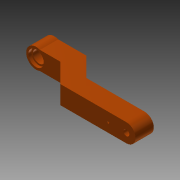
# Autodesk Inventor part: xy forearm
Saved by Autodesk Inventor 2013 (Build 170138000, 138)
## iProperties
Created: 2013-08-04
Part Number: xy forearm
Material: Generic
Document SubType Name: Modeling
Designer: employee
Density: 1 g/cm^3
Mass: 104.531 g
Surface Area: 212.692 cm^2
Volume: 104.531 cm^3
Author: employee
Autodesk Inventor part; units mm, degrees
ref_plane "YZ Plane" through (0, 0, 0) normal (1, 0, 0) x (0, 1, 0)
ref_plane "XZ Plane" through (0, 0, 0) normal (0, 1, 0) x (-1, 0, 0)
ref_plane "XY Plane" through (0, 0, 0) normal (0, 0, 1) x (1, 0, 0)
sketch "Sketch1" plane through (0, 0, 0) normal (0, 1, 0) x (-1, 0, 0)
  circle A0 centre (0, 0) radius 4.05
  line L0 (0, 12.5) -> (150, 12.5)
  arc A1 (150, -12.5) -> (150, 12.5) centre (150, 0) ccw
  line L1 (150, -12.5) -> (0, -12.5)
  arc A2 (0, 12.5) -> (0, -12.5) centre (0, 0) ccw
  dimension "d0" = 150
  dimension "d2" = 12.5
  dimension "d3" = 8.1
  constraints: 4 end point, 4 point on circle, 4 tangent, 3 centre point, 2 coincident, 1 horizontal, 1 parallel
  measures "d0" distance of A1.centre A2.centre
  measures "d2" radius of A2
  measures "d3" diameter of A0
extrude "Extrusion1" add sketch "Sketch1" along normal blind 25
sketch "Sketch2" plane through (0, 25, 0) normal (0, 1, 0) x (1, 0, 0)
  circle A0 centre (0, 0) radius 4.05 projected
  line L0 (-150, -12.5) -> (0, -12.5) projected
  line L1 (0, 12.5) -> (-150, 12.5) projected
  arc A1 (-150, 12.5) -> (-150, -12.5) centre (-150, 0) ccw projected
  line L2 (-80, 12.5) -> (-80, -12.5)
  dimension "d6" = 80
  constraints: 2 end point, 2 point on line, 1 perpendicular
  measures "d6" distance from line of A0.centre L2
extrude "Extrusion2" add sketch "Sketch2" along normal blind 26.5 contours A1 L1 L2 L0
sketch "Sketch3" plane through (-150, 0, 12.5) normal (0, 0, 1) x (1, 0, 0)
  line L0 (150, 0) -> (0, 0) projected
  line L1 (70, 25) -> (70, 51.5) projected
  line L2 (0, 51.5) -> (70, 51.5) projected
  line L3 (70, 25) -> (43.5, 51.5)
  line L4 (59.6447, 0) -> (33.1447, 26.5)
  line L5 (70, 51.5) -> (70, 25) projected
  line L6 (70, 25) -> (150, 25) projected
  line L7 (150, 0) -> (150, 25) projected
  line L8 (150, 0) -> (0, 0) projected
  line L9 (0, 0) -> (0, 51.5) projected
  line L10 (-12.5, 0) -> (-12.5, 51.5) projected
  line L11 (-12.5, 26.5) -> (33.1447, 26.5)
  line L12 (-12.5, 26.5) -> (-12.5, 0)
  line L13 (59.6447, 0) -> (-12.5, 0)
  line L14 (0, 51.5) -> (70, 51.5) projected
  dimension "d9" = 45
  dimension "d10" = 25
  dimension "d11" = 25
  constraints: 10 end point, 3 point on line, 2 collinear, 1 parallel, 1 perpendicular
  measures "d9" angle of L1 L3
  measures "d10" distance between parallel lines of L3 L4
  measures "d11" distance from line of L2.start L11
extrude "Extrusion3" cut sketch "Sketch3" against normal through all contours L0 L9 L11 L4 | L13 L10 L11 L9
sketch "Sketch4" plane through (0, 0, 12.5) normal (0, 0, 1) x (1, 0, 0)
  line L0 (-116.8553, 26.5) -> (-90.3553, 0) projected
  line L1 (-80, 25) -> (-80, 51.5) projected
  line L2 (-150, 51.5) -> (-80, 51.5) projected
  line L3 (-80, 25) -> (-106.5, 51.5)
  constraints: 2 end point, 1 parallel, 1 point on line
extrude "Extrusion4" cut sketch "Sketch4" against normal through all
sketch "Sketch5" plane through (0, 51.5, 0) normal (0, 1, 0) x (1, 0, 0)
  arc A0 (-150, 12.5) -> (-150, -12.5) centre (-150, 0) ccw projected
  circle A1 centre (-150, 0) radius 8.3
  point P0 (0, 0)
  dimension "d20" = 16.6
  constraints: 1 centre point, 1 coincident
  measures "d20" diameter of A1
extrude "Extrusion5" cut sketch "Sketch5" against normal through all
sketch "Sketch6" plane through (0, 51.5, 0) normal (0, 1, 0) x (1, 0, 0)
  circle A0 centre (-150, 0) radius 8.3 projected
  arc A1 (-150, 12.5) -> (-150, -12.5) centre (-150, 0) ccw projected
  circle A2 centre (-150, 0) radius 10.55
  point P0 (0, 0)
  dimension "d26" = 21.1
  constraints: 1 centre point, 1 coincident
  measures "d26" diameter of A2
extrude "Extrusion6" cut sketch "Sketch6" against normal blind 4
sketch "Sketch7" plane through (-150, 26.5, 12.5) normal (0, -1, 0) x (1, 0, 0)
  circle A0 centre (0, -12.5) radius 8.3 projected
  circle A1 centre (0, -12.5) radius 10.55 projected
  point P0 (150, -12.5)
extrude "Extrusion7" cut sketch "Sketch7" against normal blind 4
sketch "Sketch8" plane through (0, 51.5, 0) normal (0, 1, 0) x (1, 0, 0)
  circle A0 centre (-150, 0) radius 10.55 projected
  arc A1 (-150, 12.5) -> (-150, -12.5) centre (-150, 0) ccw projected
  circle A2 centre (-150, 0) radius 13.55
  point P0 (0, 0)
  dimension "d32" = 3
  constraints: 1 centre point, 1 coincident
  measures "d32" radial gap between concentric circles of A2 A0
extrude "Extrusion8" add sketch "Sketch8" against normal up to surface (25 mm away)
sketch "Sketch9" plane through (0, 0, 0) normal (0, -1, 0) x (1, 0, 0)
  line L0 (0, 12.5) -> (-90.3553, 12.5) projected
  circle A0 centre (0, 0) radius 4.05 projected
  line L1 (0, 0) -> (-25, 0)
  circle A1 centre (-25, 0) radius 1.5
  dimension "d35" = 25
  dimension "d36" = 3
  constraints: 2 end point, 1 centre point, 1 coincident, 1 parallel
  measures "d35" distance of L1.start L1.end
  measures "d36" diameter of A1
extrude "Extrusion9" cut sketch "Sketch9" against normal through all contours A1
sketch "Sketch14" plane through (0, 51.5, 0) normal (0, 1, 0) x (1, 0, 0)
  line L0 (-106.5, 12.5) -> (-144.77, 12.5) projected
  arc A0 (-144.77, 12.5) -> (-144.77, -12.5) centre (-150, 0) ccw projected
  line L1 (-144.77, -12.5) -> (-155.23, -12.5)
  point P0 (0, 0)
  constraints: 2 end point, 1 parallel, 1 point on circle
sketch "Sketch15" plane through (0, 51.5, 0) normal (0, 1, 0) x (1, 0, 0)
  line L0 (-106.5, 12.5) -> (-144.77, 12.5) projected
  arc A0 (-144.77, 12.5) -> (-155.23, -12.5) centre (-150, 0) ccw projected
  line L1 (-155.23, -12.5) -> (-158.4293, -12.5)
  line L2 (-158.4293, -12.5) -> (-161.7346, -6.775)
  point P0 (0, 0)
  dimension "d52" = 120
  constraints: 4 end point, 1 parallel, 1 point on circle, 1 tangent
  measures "d52" angle of L1 L2
sketch "Sketch16" plane through (0, 25, 0) normal (0, 1, 0) x (1, 0, 0)
  arc A0 (0, -12.5) -> (0, 12.5) centre (0, 0) ccw projected
  line L0 (0, 12.5) -> (-80, 12.5) projected
  line L1 (0, -12.5) -> (7.2169, -12.5)
  line L2 (7.2169, -12.5) -> (10.8253, -6.25)
  dimension "d55" = 120
  constraints: 4 end point, 2 tangent, 1 parallel, 1 point on circle
  measures "d55" angle of L2 L1
body "Solid1"
